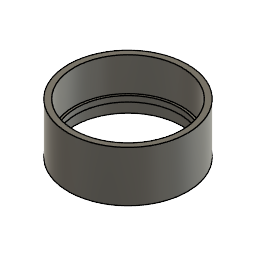
PCB CASE (Autodesk Fusion 360 design; units mm, degrees)
part number: 2026-04-27-13-45-26-943
Autodesk Fusion 360 part; units mm, degrees
sketch "Sketch1" plane through (0, 0, 0) normal (0, 1, 0) x (1, 0, 0)
  circle A0 centre (0, 0) radius 48
  circle A1 centre (0, 0) radius 53
  dimension "d1" = 96
  dimension "d2" = 106
  constraint coincident A0.centre A1.centre
  constraint concentric A0 A1
  measures "d1" diameter of A0
  measures "d2" diameter of A1
extrude "Extrude1" add sketch "Sketch1" along normal blind 30
sketch "Sketch2" plane through (0, 0, 0) normal (0, -1, 0) x (1, 0, 0)
  circle A0 centre (0, 0) radius 48
  circle A1 centre (0, 0) radius 53
  circle A2 centre (0, 0) radius 46
  dimension "d5" = 92
  constraint coincident A0.centre A1.centre
  measures "d5" diameter of A2
extrude "Extrude2" add sketch "Sketch2" along normal blind 5 contours A0 | A1
sketch "Sketch3" plane through (0, -5, 0) normal (0, -1, 0) x (1, 0, 0)
  circle A0 centre (0, 0) radius 46
  circle A1 centre (0, 0) radius 53
  circle A2 centre (0, 0) radius 48
  dimension "d8" = 96
  constraint coincident A0.centre A1.centre
  measures "d8" diameter of A2
extrude "Extrude3" add sketch "Sketch3" along normal blind 10 contours A1
